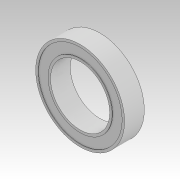
# Autodesk Inventor part: 6701 bearing
Saved by Autodesk Inventor 2020 (Build 240168000, 168)
## iProperties
Created: 2020-11-25
Part Number: 6701 bearing
Material: Generic
Document SubType Name: Modeling
Designer: DDeGo
Density: 1 g/cm^3
Appearance: Default
Author: DDeGo
Autodesk Inventor part; units mm, degrees
ref_plane "YZ Plane" through (0, 0, 0) normal (1, 0, 0) x (0, 1, 0)
ref_plane "XZ Plane" through (0, 0, 0) normal (0, 1, 0) x (-1, 0, 0)
ref_plane "XY Plane" through (0, 0, 0) normal (0, 0, 1) x (1, 0, 0)
sketch "Sketch1" plane through (0, 0, 0) normal (1, 0, 0) x (0, 1, 0)
  line L0 (0, 0) -> (0, -2.1848) construction
  line L1 (0, 0) -> (6, 0) construction
  line L2 (6, 0) -> (6, -2)
  line L3 (6, -2) -> (6.5, -2)
  line L4 (6.5, -2) -> (6.5, -1.9)
  line L5 (6.5, -1.9) -> (8.5, -1.9)
  line L6 (8.5, -1.9) -> (8.5, -2)
  line L7 (8.5, -2) -> (9, -2)
  line L8 (9, -2) -> (9, 0)
  line L9 (9, 0) -> (6, 0) construction
  line L10 (6, 0) -> (6, 2)
  line L11 (6, 2) -> (6.5, 2)
  line L12 (6.5, 2) -> (6.5, 1.9)
  line L13 (6.5, 1.9) -> (8.5, 1.9)
  line L14 (8.5, 1.9) -> (8.5, 2)
  line L15 (8.5, 2) -> (9, 2)
  line L16 (9, 2) -> (9, 0)
  dimension "d0" = 6
  dimension "d1" = 9
  dimension "d2" = 0.1
  dimension "d3" = 2
  dimension "d6" = 4
  constraints: 34 end point, 7 perpendicular, 6 symmetric about line, 5 point on line, 1 collinear, 1 horizontal, 1 vertical
  measures "d0" distance between parallel lines of L0 L2
  measures "d1" distance between parallel lines of L0 L8
  measures "d2" distance between parallel lines of L7 L5
  measures "d3" distance of L4.end L5.end
  measures "d6" distance between parallel lines of L3 L11
revolve "Revolution1" add sketch "Sketch1" angle 360 about axis through (0, 0, 0) along (0, 0, -1)
body "Solid1"
